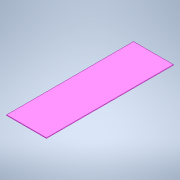
# Autodesk Inventor part: Base
Saved by Autodesk Inventor 2021 (Build 250183000, 183)
## iProperties
Created: 2022-02-04
Part Number: Base
Material: Generic
Document SubType Name: Modeling
Designer: tlar613
Density: 1 g/cm^3
Appearance: Default
Author: tlar613
Autodesk Inventor part; units mm, degrees
ref_plane "YZ Plane" through (0, 0, 0) normal (1, 0, 0) x (0, 1, 0)
ref_plane "XZ Plane" through (0, 0, 0) normal (0, 1, 0) x (-1, 0, 0)
ref_plane "XY Plane" through (0, 0, 0) normal (0, 0, 1) x (1, 0, 0)
sketch "Sketch1" plane through (0, 0, 0) normal (0, 1, 0) x (-1, 0, 0)
  line L0 (160, 510) -> (-160, 510)
  line L1 (-160, 510) -> (-160, -510)
  line L2 (-160, -510) -> (160, -510)
  line L3 (160, -510) -> (160, 510)
  line L4 (0, -714) -> (0, 714) projected
  line L5 (-224, 0) -> (224, 0) projected
  point P0 (0, 0)
  dimension "d0" = 1020
  dimension "d1" = 320
  constraints: 8 end point, 2 parallel, 1 horizontal, 1 perpendicular, 2 other
  measures "d0" distance of L2.end L0.start
  measures "d1" distance of L1.end L2.end
extrude "Extrusion1" add sketch "Sketch1" along normal blind 5
body "Solid1"
